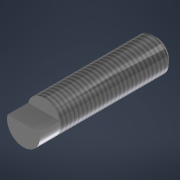
# Autodesk Inventor part: Tornillo de elevación
Saved by Autodesk Inventor 2022 (Build 260153000, 153)
## iProperties
Created: 2021-09-10
Part Number: Tornillo de elevación
Material: Stainless Steel, 440C
Document SubType Name: Modeling
Designer: Andres
Density: 7.75 g/cm^3
Appearance: Semi-Polished
Author: Andres
Autodesk Inventor part; units mm, degrees
ref_plane "YZ Plane" through (0, 0, 0) normal (1, 0, 0) x (0, 1, 0)
ref_plane "XZ Plane" through (0, 0, 0) normal (0, 1, 0) x (-1, 0, 0)
ref_plane "XY Plane" through (0, 0, 0) normal (0, 0, 1) x (1, 0, 0)
sketch "Sketch1" plane through (0, 0, 0) normal (0, 0, 1) x (1, 0, 0)
  circle A0 centre (0, 0) radius 8
  dimension "d0" = 16
  constraints: 1 centre point, 1 coincident
  measures "d0" diameter of A0
extrude "Extrusion1" add sketch "Sketch1" along normal blind 55
thread "Thread1" size "TR16x2" class "7e" standard "ISO Metric Trapezoidal Threads" length 55
sketch "Sketch2" plane through (0, 0, 55) normal (0, 0, 1) x (1, 0, 0)
  circle A0 centre (0, 0) radius 8 projected
  circle A1 centre (0, 0) radius 8 projected
  line L0 (7.746, 2) -> (-7.746, 2)
  dimension "d20" = 2
  constraints: 2 end point, 2 point on circle, 1 horizontal
  measures "d20" distance from line of L0 point (0, 0)
extrude "Extrusion2" add sketch "Sketch2" along normal blind 10 contours A0 L0 picked at (-0.9989, -2.013)
chamfer "Chamfer1" distance 2 angle 45 1 edges at (-8, 0, 0)
sketch "Sketch4" plane through (0, 0, 0) normal (0, 1, 0) x (-1, 0, 0)
  line L0 (7.746, 65) -> (-7.746, 65) projected
  line L1 (-8, 2) -> (8, 2) projected
  line L2 (0, 57) -> (0, 63) construction
  line L3 (1.5, 57) -> (1.5, 63)
  line L4 (-1.5, 63) -> (-1.5, 57)
  arc A0 (-1.5, 57) -> (1.5, 57) centre (0, 57) ccw
  arc A1 (1.5, 63) -> (-1.5, 63) centre (0, 63) ccw
  line L5 (-7.746, 55) -> (-7.746, 65) projected
  line L6 (7.746, 55) -> (7.746, 65) projected
  line L7 (-7.746, 55) -> (7.746, 55) projected
  point P0 (0, 0)
  point P1 (8, 65)
  point P2 (-8, 65)
  point P3 (0, 60)
  point P4 (1.5, 63)
  point P5 (0, 65)
  dimension "d13" = 3
  dimension "d14" = 3
  dimension "d19" = 5
  constraints: 8 end point, 4 point on circle, 4 tangent, 2 centre point, 2 midpoint, 1 parallel, 1 vertical, 1 vertical alignment
  measures "d13" distance of point (0, 60) L2.end
  measures "d14" diameter of A1
  measures "d19" distance from line of L0 point (0, 60)
extrude "Extrusion3" [suppressed]
extrude "Extrusion4" [suppressed]
body "Solid1"
